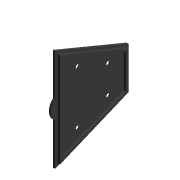
# Autodesk Inventor part: Modul Deckel
Saved by Autodesk Inventor 2018.2 (Build 222227000, 227)
## iProperties
Created: 2018-10-15
Part Number: Modul Deckel
Material: PC/ABS-Kunststoff
Document SubType Name: Modeling
Designer: N.Grubert
Density: 0.357273 g/cm^3
Appearance: Glatt - weiß
Mass: 7.73118 g
Surface Area: 180.305 cm^2
Volume: 21.6394 cm^3
Fläche: 0 cm²
Gewicht: 0 g
Material: geeigneten Werkstoff auswählen !
Dateiname: P:\INVENTOR\Inventor 2018\Templates\ILT\Norm.ipt
Bez_eng: bolt
Bez_french: boulon
Author: N.Grubert
Autodesk Inventor part; units mm, degrees
ref_plane "YZ Plane" through (0, 0, 0) normal (1, 0, 0) x (0, 1, 0)
ref_plane "XZ Plane" through (0, 0, 0) normal (0, 1, 0) x (-1, 0, 0)
ref_plane "XY Plane" through (0, 0, 0) normal (0, 0, 1) x (1, 0, 0)
sketch "Skizze4" plane through (0, 0, 0) normal (1, 0, 0) x (0, 1, 0)
  line L0 (44.5, 24.853) -> (-44.5, 61.718)
  line L1 (-44.5, 61.718) -> (-44.5, -61.718)
  line L2 (-44.5, -61.718) -> (44.5, -24.853)
  line L3 (44.5, -24.853) -> (44.5, 24.853)
  line L4 (0, -86.4052) -> (0, 86.4052) construction
  line L5 (-62.3, 0) -> (62.3, 0) construction
  dimension "d34" = 89
  dimension "d37" = 112.5
  dimension "d38" = 49.706
  constraints: 8 end point, 2 parallel, 2 other
  measures "d34" distance between parallel lines of L3 L1
  measures "d37" angle of L0 L3
  measures "d38" distance of L2.end L0.start
extrude "Extrusion2" add sketch "Skizze4" along normal blind 2.5
sketch "Skizze5" plane through (2.5, 0, 0) normal (1, 0, 0) x (0, 0, -1)
  line L0 (-61.718, -44.5) -> (61.718, -44.5) construction
  line L1 (61.718, -44.5) -> (24.853, 44.5) construction
  line L2 (24.853, 44.5) -> (-24.853, 44.5) construction
  line L3 (-24.853, 44.5) -> (-61.718, -44.5) construction
  line L4 (-22.8485, 41.5) -> (22.8485, 41.5)
  line L5 (22.8485, 41.5) -> (57.2282, -41.5)
  line L6 (57.2282, -41.5) -> (-57.2282, -41.5)
  line L7 (-57.2282, -41.5) -> (-22.8485, 41.5)
  line L8 (20.8439, 38.5) -> (-20.8439, 38.5)
  line L9 (-20.8439, 38.5) -> (-52.7384, -38.5)
  line L10 (-52.7384, -38.5) -> (52.7384, -38.5)
  line L11 (52.7384, -38.5) -> (20.8439, 38.5)
  point P0 (0, 0)
  dimension "d8" = 3
  dimension "d9" = 3
  constraints: 16 end point, 6 other
  measures "d8" distance between parallel lines of L2 L4
  measures "d9" distance between parallel lines of L4 L8
extrude "Extrusion3" add sketch "Skizze5" along normal blind 3
sketch "Skizze6" plane through (0, 0, 0) normal (-1, 0, 0) x (0, 0, 1)
  line L0 (24.853, 44.5) -> (-24.853, 44.5) construction
  line L1 (61.718, -44.5) -> (24.853, 44.5) construction
  line L2 (-24.853, 44.5) -> (24.853, 44.5) projected
  line L3 (0, 57.3) -> (0, -53.3) construction
  line L4 (-61.718, -44.5) -> (61.718, -44.5) construction
  arc A0 (-11.1803, -44.5) -> (11.1803, -44.5) centre (0, -34.5) ccw
  line L5 (-11.1803, -44.5) -> (11.1803, -44.5)
  dimension "d35" = 15
  dimension "d36" = 10
  constraints: 4 end point, 3 point on line, 2 point on circle, 1 centre point, 1 horizontal, 1 vertical, 2 other
  measures "d35" radius of A0
  measures "d36" distance from line of L4 A0.centre
extrude "Extrusion4" add sketch "Skizze6" against normal up to surface (2.5 mm away)
sketch "Skizze8" plane through (0, 0, 0) normal (-1, 0, 0) x (0, 0, 1)
  circle A0 centre (0, 56.5) radius 2 construction
  line L0 (-61.718, -44.5) -> (-11.1803, -44.5) construction
  arc A1 (-11.1803, -44.5) -> (11.1803, -44.5) centre (0, -34.5) ccw construction
  line L1 (11.1803, -44.5) -> (61.718, -44.5) construction
  line L2 (61.718, -44.5) -> (24.853, 44.5) construction
  line L3 (24.853, 44.5) -> (-24.853, 44.5) construction
  line L4 (-24.853, 44.5) -> (-61.718, -44.5) construction
  line L5 (0, -71.1) -> (0, 80.1) construction
  line L6 (-86.4052, 0) -> (86.4052, 0) construction
  line L7 (-16.8941, 19.5) -> (16.8941, 19.5) construction
  line L8 (-32.22, -17.5) -> (32.22, -17.5) construction
  line L9 (32.22, -17.5) -> (16.8941, 19.5) construction
  line L10 (-16.8941, 19.5) -> (-32.22, -17.5) construction
  point P0 (0, 0)
  dimension "d42" = 37
  dimension "d53" = 112.5
  dimension "d54" = 25
  constraints: 8 end point, 2 coincident, 1 horizontal, 1 parallel, 1 other
  measures "d42" distance between parallel lines of L8 L7
  measures "d53" angle of L3 L9
  measures "d54" distance between parallel lines of L7 L3
hole "Bohrung2" at (0, 19.5, -16.8941) at (0, -17.5, -32.22) at (0, -17.5, 32.22) at (0, 19.5, 16.8941) direction (1, 0, 0) diameter 4 end through all
chamfer "Fase2" distance 2 angle 45 4 edges at (0, 19.5, -18.8941) (0, 19.5, 14.8941) (0, -17.5, -34.22) (0, -17.5, 30.22)
